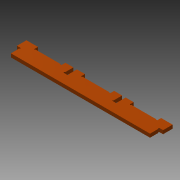
# Autodesk Inventor part: shortSlat
Saved by Autodesk Inventor 2015 SP1 (Build 190203100, 203)
## iProperties
Created: 2015-04-09
Part Number: shortSlat
Material: Generic
Document SubType Name: Modeling
Designer: Iain
Density: 1 g/cm^3
Appearance: Smooth - Light Orange
Author: Iain
Autodesk Inventor part; units mm, degrees
ref_plane "YZ Plane" through (0, 0, 0) normal (1, 0, 0) x (0, 1, 0)
sketch "Sketch1" plane through (0, 0, 0) normal (0, 0, 1) x (1, 0, 0)
  line L0 (-375, 40) -> (375, 40)
  line L1 (375, 40) -> (375, -40)
  line L2 (375, -40) -> (-375, -40)
  line L3 (-375, -40) -> (-375, 40)
  point P0 (0, 0)
  point P1 (375, 0)
  point P2 (0, 40)
  dimension "d0" = 750
  dimension "d1" = 80
  constraints: 8 end point, 2 midpoint, 2 parallel, 1 horizontal, 1 horizontal alignment, 1 perpendicular, 1 vertical alignment
  measures "d0" distance of L0.start L0.end
  measures "d1" distance of L2.end L0.start
extrude "Extrusion1" add sketch "Sketch1" along normal blind 18
sketch "Sketch2" plane through (0, 0, 18) normal (0, 0, 1) x (1, 0, 0)
  line L0 (375, 40) -> (-375, 40) projected
  line L1 (-375, 40) -> (-375, -40) projected
  line L2 (-375, -40) -> (375, -40) projected
  line L3 (375, -40) -> (375, 40) projected
  line L4 (-375, 58) -> (-316, 58)
  line L5 (-316, 58) -> (-316, 40)
  line L6 (-316, 40) -> (-375, 40)
  line L7 (-375, 40) -> (-375, 58)
  point P0 (0, 0)
  point P1 (-345.5, 40)
  point P2 (0, 40)
  point P3 (-375, 49)
  point P4 (-375, 0)
  dimension "d4" = 18
  dimension "d5" = 59
  constraints: 8 end point, 4 midpoint, 2 parallel, 1 horizontal, 1 horizontal alignment, 1 perpendicular, 1 vertical alignment
  measures "d4" distance of L4.end L5.end
  measures "d5" distance of L4.start L4.end
extrude "Extrusion2" add sketch "Sketch2" against normal blind 18 contours L0 L7 L4 L5
sketch "Sketch3" plane through (0, 0, 18) normal (0, 0, 1) x (1, 0, 0)
  line L0 (-175, 58) -> (-75, 58)
  line L1 (-75, 58) -> (-75, 40)
  line L2 (-75, 40) -> (-175, 40)
  line L3 (-175, 40) -> (-175, 58)
  line L4 (375, 40) -> (-316, 40) projected
  line L5 (-316, 58) -> (-316, 40) projected
  line L6 (-375, 58) -> (-316, 58) projected
  line L7 (-375, -40) -> (-375, 58) projected
  line L8 (-375, -40) -> (375, -40) projected
  line L9 (375, -40) -> (375, 40) projected
  point P0 (0, 0)
  point P1 (-125, 40)
  point P2 (29.5, 40)
  dimension "d8" = 100
  dimension "d9" = 18
  dimension "d10" = 250
  constraints: 8 end point, 2 midpoint, 2 parallel, 1 horizontal, 1 horizontal alignment, 1 perpendicular
  measures "d8" distance of L0.start L0.end
  measures "d9" distance of L0.end L1.end
  measures "d10" distance from line of L7 point (-125, 40)
extrude "Extrusion3" add sketch "Sketch3" against normal blind 18 contours L0 L1 L2 L3
sketch "Sketch4" plane through (0, 0, 18) normal (0, 0, 1) x (1, 0, 0)
  line L0 (375, 40) -> (-75, 40) projected
  line L1 (-75, 58) -> (-75, 40) projected
  line L2 (-175, 58) -> (-75, 58) projected
  line L3 (-175, 40) -> (-175, 58) projected
  line L4 (-175, 40) -> (-316, 40) projected
  line L5 (-316, 58) -> (-316, 40) projected
  line L6 (-375, 58) -> (-316, 58) projected
  line L7 (-375, -40) -> (-375, 58) projected
  line L8 (-375, -40) -> (375, -40) projected
  line L9 (375, -40) -> (375, 40) projected
  line L10 (-375, -40) -> (-357, -40)
  line L11 (-357, -40) -> (-357, 9)
  line L12 (-357, 9) -> (-375, 9)
  line L13 (-375, 9) -> (-375, -40)
  point P0 (0, 0)
  point P1 (-366, -40)
  point P2 (0, -40)
  point P3 (-375, -15.5)
  point P4 (-375, 9)
  dimension "d13" = 18
  dimension "d14" = 49
  constraints: 8 end point, 4 midpoint, 2 parallel, 1 horizontal, 1 horizontal alignment, 1 perpendicular, 1 vertical alignment
  measures "d13" distance of L11.end L12.end
  measures "d14" distance of L10.end L11.end
extrude "Extrusion4" cut sketch "Sketch4" against normal blind 18 contours L8 L7 L12 L11
sketch "Sketch5" plane through (0, 0, 18) normal (0, 0, 1) x (1, 0, 0)
  line L0 (-134, 58) -> (-116, 58)
  line L1 (-116, 58) -> (-116, 9)
  line L2 (-116, 9) -> (-134, 9)
  line L3 (-134, 9) -> (-134, 58)
  line L4 (-375, 9) -> (-357, 9) projected
  line L5 (-357, 9) -> (-357, -40) projected
  line L6 (-357, -40) -> (375, -40) projected
  line L7 (375, -40) -> (375, 40) projected
  line L8 (375, 40) -> (-75, 40) projected
  line L9 (-75, 58) -> (-75, 40) projected
  line L10 (-175, 58) -> (-75, 58) projected
  line L11 (-175, 40) -> (-175, 58) projected
  line L12 (-175, 40) -> (-316, 40) projected
  line L13 (-316, 58) -> (-316, 40) projected
  line L14 (-375, 58) -> (-316, 58) projected
  line L15 (-375, 9) -> (-375, 58) projected
  line L16 (-175, 58) -> (-75, 58) projected
  point P0 (0, 0)
  point P1 (-125, 58)
  point P2 (-125, 58)
  point P3 (-125, 58)
  dimension "d17" = 18
  dimension "d18" = 49
  constraints: 8 end point, 3 midpoint, 2 coincident, 2 parallel, 1 horizontal, 1 perpendicular
  measures "d17" distance of L0.start L0.end
  measures "d18" distance of L0.end L1.end
extrude "Extrusion5" cut sketch "Sketch5" against normal blind 18 contours L0 L1 L2 L3
ref_plane "Work Plane1" through (0, 58, 0) normal (-1, 0, 0) x (0, 0, 1)
mirror "Mirror1" about plane through (0, 58, 0) normal (-1, 0, 0) of "Extrusion5", "Extrusion4", "Extrusion3", "Extrusion2"
sketch "Sketch6" plane through (0, 0, 18) normal (0, 0, 1) x (1, 0, 0)
  line L0 (357, 9) -> (375, 9) projected
  line L1 (375, 9) -> (375, 58) projected
  line L2 (375, 58) -> (316, 58) projected
  line L3 (316, 58) -> (316, 40) projected
  line L4 (316, 40) -> (175, 40) projected
  line L5 (175, 40) -> (175, 58) projected
  line L6 (175, 58) -> (134, 58) projected
  line L7 (134, 58) -> (134, 9) projected
  line L8 (134, 9) -> (116, 9) projected
  line L9 (116, 9) -> (116, 58) projected
  line L10 (116, 58) -> (75, 58) projected
  line L11 (75, 58) -> (75, 40) projected
  line L12 (75, 40) -> (-75, 40) projected
  line L13 (-75, 58) -> (-75, 40) projected
  line L14 (-116, 58) -> (-75, 58) projected
  line L15 (-116, 58) -> (-116, 9) projected
  line L16 (-116, 9) -> (-134, 9) projected
  line L17 (-134, 9) -> (-134, 58) projected
  line L18 (-175, 58) -> (-134, 58) projected
  line L19 (-175, 40) -> (-175, 58) projected
  line L20 (-175, 40) -> (-316, 40) projected
  line L21 (-316, 58) -> (-316, 40) projected
  line L22 (-375, 58) -> (-316, 58) projected
  line L23 (-375, 9) -> (-375, 58) projected
  line L24 (-375, 9) -> (-357, 9) projected
  line L25 (-357, 9) -> (-357, -40) projected
  line L26 (-357, -40) -> (357, -40) projected
  line L27 (357, -40) -> (357, 9) projected
  point P0 (0, 0)
  point P1 (-357, 5.825)
  point P2 (-312.825, 40)
  dimension "d21" = 3.175
  dimension "d22" = 3.175
  constraints: 1 horizontal alignment, 1 vertical alignment
  measures "d21" distance from line of L24 point (-357, 5.825)
  measures "d22" distance from line of L21 point (-312.825, 40)
hole "Hole1" at (-357, 5.825, 18) at (-312.825, 40, 18) direction (0, 0, -1) diameter 6.35 end through all
mirror "Mirror2" about plane through (0, 58, 0) normal (-1, 0, 0) of "Hole1"
sketch "Sketch7" plane through (0, 0, 18) normal (0, 0, 1) x (1, 0, 0)
  arc A0 (357, 9) -> (357, 2.65) centre (357, 5.825) ccw projected
  line L0 (357, 9) -> (375, 9) projected
  line L1 (375, 9) -> (375, 58) projected
  line L2 (375, 58) -> (316, 58) projected
  line L3 (316, 58) -> (316, 40) projected
  arc A1 (309.65, 40) -> (316, 40) centre (312.825, 40) ccw projected
  line L4 (309.65, 40) -> (175, 40) projected
  line L5 (175, 40) -> (175, 58) projected
  line L6 (175, 58) -> (134, 58) projected
  line L7 (134, 58) -> (134, 9) projected
  line L8 (134, 9) -> (116, 9) projected
  line L9 (116, 9) -> (116, 58) projected
  line L10 (116, 58) -> (75, 58) projected
  line L11 (75, 58) -> (75, 40) projected
  line L12 (75, 40) -> (-75, 40) projected
  line L13 (-75, 58) -> (-75, 40) projected
  line L14 (-116, 58) -> (-75, 58) projected
  line L15 (-116, 58) -> (-116, 9) projected
  line L16 (-116, 9) -> (-134, 9) projected
  line L17 (-134, 9) -> (-134, 58) projected
  line L18 (-175, 58) -> (-134, 58) projected
  line L19 (-175, 40) -> (-175, 58) projected
  line L20 (-175, 40) -> (-309.65, 40) projected
  arc A2 (-316, 40) -> (-309.65, 40) centre (-312.825, 40) ccw projected
  line L21 (-316, 58) -> (-316, 40) projected
  line L22 (-375, 58) -> (-316, 58) projected
  line L23 (-375, 9) -> (-375, 58) projected
  line L24 (-375, 9) -> (-357, 9) projected
  arc A3 (-357, 2.65) -> (-357, 9) centre (-357, 5.825) ccw projected
  line L25 (-357, 2.65) -> (-357, -40) projected
  line L26 (-357, -40) -> (357, -40) projected
  line L27 (357, -40) -> (357, 2.65) projected
  point P0 (0, 0)
  point P1 (-178.175, 40)
  point P2 (-134, 12.175)
  point P3 (-242.325, 40)
  dimension "d30" = 3.175
  dimension "d31" = 3.175
  constraints: 1 horizontal alignment, 1 midpoint, 1 vertical alignment
  measures "d30" distance from line of L19 point (-178.175, 40)
  measures "d31" distance from line of L16 point (-134, 12.175)
hole "Hole2" at (-178.175, 40, 18) at (-134, 12.175, 18) direction (0, 0, -1) diameter 6.35 end through all
ref_plane "Work Plane2" through (-125, 58, 18) normal (1, 0, 0) x (0, 0, -1)
mirror "Mirror3" about plane through (-125, 58, 18) normal (1, 0, 0) of "Hole2"
mirror "Mirror4" about plane through (0, 58, 0) normal (-1, 0, 0) of "Hole2", "Mirror3"
equation "\"d0\" = tableWidth"
equation "\"d1\" = legTopDepth"
equation "\"d2\" = plyThickness"
equation "\"d4\" = legTopTabHeight"
equation "\"d5\" = 0.5 * plyThickness + 0.5 * legTabTotalWidth"
equation "\"d6\" = plyThickness"
equation "\"d8\" = legTabTotalWidth"
equation "\"d9\" = legTopTabHeight"
equation "\"d10\" = 0.333333 * tableWidth"
equation "\"d11\" = plyThickness"
equation "\"d13\" = plyThickness"
equation "\"d14\" = legTopSlotDepth"
equation "\"d15\" = plyThickness"
equation "\"d17\" = plyThickness"
equation "\"d18\" = legTopSlotDepth"
equation "\"d19\" = plyThickness"
equation "\"d21\" = 0.5 * millDiameter"
equation "\"d22\" = 0.5 * millDiameter"
equation "\"d23\" = millDiameter"
equation "\"d30\" = 0.5 * millDiameter"
equation "\"d31\" = 0.5 * millDiameter"
equation "\"d32\" = millDiameter"
equation "\"plyThickness\" = 18"
equation "\"legHeight\" = 702"
equation "\"tableWidth\" = 750"
equation "\"legTopDepth\" = 80"
equation "\"millDiameter\" = 6.35"
equation "\"legTopTabHeight\" = 18"
equation "\"legTabTotalWidth\" = 100"
equation "\"legTopSlotDepth\" = 49"
body "Solid1"
